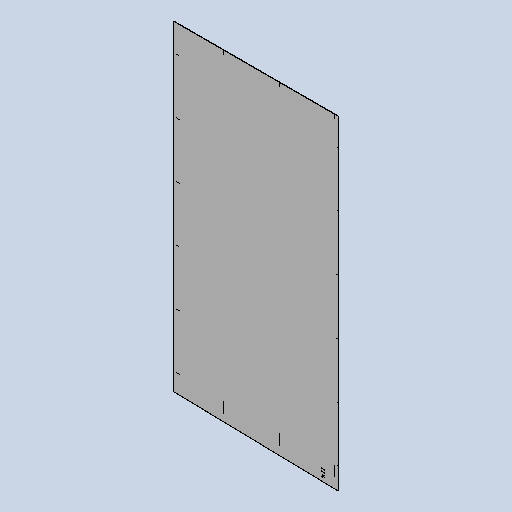
# Autodesk Inventor part: GBK 2211 shield 4
Saved by Autodesk Inventor 2026.2 (Build 302298010, 298A)
## iProperties
Created: 2026-04-17
Part Number: GBK 2211 shield 4
Material: Steel
Document SubType Name: Sheet Metal
Designer: pokla
Stock Number: 2214
Mass: 138487 g
Surface Area: 88564.8 cm^2
Volume: 17641.6 cm^3
Density: 7.85 g/cm^3
Flat Pattern Width: 148 cm
Flat Pattern Length: 292 cm
Flat Pattern Area: 43216 cm^2
Sheet Metal Rule: Default_mm
Sheet Metal Width: 1480,000 mm
Sheet Metal Length: 2920,000 mm
Sheet Metal Area: 4321600,000 mm^2
Appearance: Default
Author: admin
Autodesk Inventor part; units mm, degrees
ref_plane "YZ Plane" through (0, 0, 0) normal (1, 0, 0) x (0, 1, 0)
ref_plane "XZ Plane" through (0, 0, 0) normal (0, 1, 0) x (-1, 0, 0)
ref_plane "XY Plane" through (0, 0, 0) normal (0, 0, 1) x (1, 0, 0)
sketch "Sketch1" plane through (0, 0, 0) normal (0, 0, 1) x (1, 0, 0)
  line L0 (740, -1490) -> (-740, -1490)
  line L1 (-740, -1490) -> (-740, 1490)
  line L2 (-740, 1490) -> (740, 1490)
  line L3 (740, 1490) -> (740, -1490)
  line L4 (740, -1490) -> (-740, 1490) construction
  line L5 (-740, -1490) -> (740, 1490) construction
  line L6 (740, -1430) -> (-740, -1396.4141)
  point P0 (0, 0)
  dimension "d0" = 1480
  dimension "d1" = 2980
  dimension "d3" = 1.3
  dimension "d4" = 60
  measures "d0" distance of L1.end L2.end
  measures "d1" distance of L0.end L1.end
  measures "d3" angle of L0 L6
  measures "d4" distance of L0.start L6.start
extrude "Plate1" add sketch "Sketch1" along normal blind 4 contours L6 L1 L2 L3
sketch "Sketch2" plane through (0, 0, 4) normal (0, 0, 1) x (1, 0, 0)
  line L0 (621.6658, -1316.5027) -> (621.6658, -1674.1932) construction
  line L1 (621.6658, -1674.1932) -> (530.4095, -1674.1932) construction
  line L2 (530.4095, -1674.1932) -> (530.4095, -1316.5027) construction
  line L3 (530.4095, -1316.5027) -> (621.6658, -1316.5027) construction
  line L4 (790.0856, -1236) -> (730.0856, -1236) projected
  line L5 (730.0856, -1240) -> (730.0856, -1236) projected
  line L6 (710.3341, -1243.5) -> (710.3341, -1340.5) projected
  line L7 (710.3341, -1340.5) -> (706.3352, -1340.5) projected
  ellipse E0 centre (710.3341, 1484.5) end of major axis (710.3341, 1514.5) minor radius 0.6803 (710.3341, 1454.5) -> (710.3341, 1514.5) ccw projected
  line L8 (710.3341, 1454.5) -> (706.3352, 1454.5) projected
  line L9 (790.0856, 1247.3333) -> (730.0856, 1247.3333) projected
  line L10 (730.0856, 1243.3333) -> (730.0856, 1247.3333) projected
  line L11 (790.0856, 750.6667) -> (730.0856, 750.6667) projected
  line L12 (730.0856, 746.6667) -> (730.0856, 750.6667) projected
  line L13 (790.0856, 254) -> (730.0856, 254) projected
  line L14 (730.0856, 250) -> (730.0856, 254) projected
  line L15 (790.0856, -242.6667) -> (730.0856, -242.6667) projected
  line L16 (730.0856, -246.6667) -> (730.0856, -242.6667) projected
  line L17 (790.0856, -739.3333) -> (730.0856, -739.3333) projected
  line L18 (730.0856, -743.3333) -> (730.0856, -739.3333) projected
  ellipse E1 centre (210.2055, 1484.5) end of major axis (210.2055, 1514.5) minor radius 0.6803 (210.2055, 1454.5) -> (210.2055, 1514.5) ccw projected
  line L19 (210.2055, 1454.5) -> (206.2066, 1454.5) projected
  ellipse E2 centre (-289.9231, 1484.5) end of major axis (-289.9231, 1514.5) minor radius 0.6803 (-289.9231, 1454.5) -> (-289.9231, 1514.5) ccw projected
  line L20 (-289.9231, 1454.5) -> (-293.922, 1454.5) projected
  line L21 (-689.9144, 1247.3333) -> (-719.2342, 1247.3333) projected
  line L22 (-689.9144, 1243.3333) -> (-689.9144, 1247.3333) projected
  line L23 (-689.9144, 750.6667) -> (-719.2342, 750.6667) projected
  line L24 (-689.9144, 746.6667) -> (-689.9144, 750.6667) projected
  line L25 (-689.9144, 254) -> (-719.2342, 254) projected
  line L26 (-689.9144, 250) -> (-689.9144, 254) projected
  line L27 (-689.9144, -242.6667) -> (-719.2342, -242.6667) projected
  line L28 (-689.9144, -246.6667) -> (-689.9144, -242.6667) projected
  line L29 (-689.9144, -739.3333) -> (-719.2342, -739.3333) projected
  line L30 (-689.9144, -743.3333) -> (-689.9144, -739.3333) projected
  line L31 (-689.9144, -1236) -> (-719.2342, -1236) projected
  line L32 (-689.9144, -1240) -> (-689.9144, -1236) projected
  line L33 (-289.9231, -1243.5) -> (-289.9231, -1340.5) projected
  line L34 (-289.9231, -1340.5) -> (-293.922, -1340.5) projected
  line L35 (210.2055, -1243.5) -> (210.2055, -1340.5) projected
  line L36 (210.2055, -1340.5) -> (206.2066, -1340.5) projected
  point P0 (0, 0)
  constraints: 5 other
mark "Mark1"
equation "\"d0\" = Лист_ширина"
equation "\"d2\" = Thickness"
equation "\"BendRadius\" = Thickness"
equation "\"BendReliefWidth\" = Thickness"
equation "\"BendReliefDepth\" = 0.5 * Thickness"
equation "\"CornerReliefSize\" = 4 * Thickness"
equation "\"MinimumRemnant\" = 2 * Thickness"
equation "\"TransitionRadius\" = BendRadius"
equation "\"JacobiRadiusSize\" = BendRadius"
equation "\"GapSize\" = Thickness"
equation "\"Лист_ширина\" = 1480"
equation "\"Thickness\" = 4"
body "Solid1"
